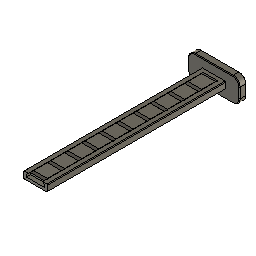
Price Tracker Final (Autodesk Fusion 360 design; units mm, degrees)
Autodesk Fusion 360 part; units mm, degrees
sketch "Sketch1" plane through (0, 0, 0) normal (0, 0, 1) x (1, 0, 0)
  line L0 (12.5, -12.5) -> (-12.5, -12.5)
  line L1 (-12.5, -12.5) -> (-12.5, 12.5)
  line L2 (-12.5, 12.5) -> (12.5, 12.5)
  line L3 (12.5, 12.5) -> (12.5, -12.5)
  line L4 (12.5, -12.5) -> (-12.5, 12.5) construction
  line L5 (-12.5, -12.5) -> (12.5, 12.5) construction
  dimension "d1" = 25
  dimension "d2" = 25
  constraint horizontal L0
  constraint perpendicular L0 L1
  constraint parallel L0 L2
  constraint parallel L1 L3
  constraint coincident L4 origin
  constraint coincident L5 origin
  measures "d1" distance of L1.end L2.end
  measures "d2" distance of L0.end L1.end
extrude "Extrude1" add sketch "Sketch1" along normal blind 5 makes body 1
chamfer "Chamfer1" distance 2.5 angle 45 1 faces at (4.1667, -4.1667, 5) on bodies 1
pattern_linear "R-Pattern1" count 10 spacing 25 along (0, 1, 0) of bodies 1 makes body 2 at (4.1667, 20.8333, 0) makes body 3 at (4.1667, 45.8333, 0) makes body 4 at (4.1667, 70.8333, 0) makes body 5 at (4.1667, 95.8333, 0) makes body 6 at (4.1667, 120.8333, 0) makes body 7 at (4.1667, 145.8333, 0) makes body 8 at (4.1667, 170.8333, 0) makes body 9 at (4.1667, 195.8333, 0) makes body 10 at (4.1667, 220.8333, 0)
sketch "Sketch2" plane through (0, 0, 0) normal (0, 0, 1) x (1, 0, 0)
  line L0 (17.5, 242.5) -> (-17.5, 242.5)
  line L1 (-17.5, 242.5) -> (-17.5, -17.5)
  line L2 (-17.5, -17.5) -> (17.5, -17.5)
  line L3 (17.5, -17.5) -> (17.5, 242.5)
  line L4 (17.5, 242.5) -> (-17.5, -17.5) construction
  line L5 (-17.5, 242.5) -> (17.5, -17.5) construction
  line L6 (-12.5, 12.5) -> (12.5, 12.5) construction
  line L7 (12.5, 12.5) -> (12.5, -12.5) construction
  line L8 (12.5, -12.5) -> (-12.5, -12.5) construction
  line L9 (-12.5, -12.5) -> (-12.5, 12.5) construction
  line L10 (-17.5, -17.5) -> (-17.5, 17.5)
  line L11 (-17.5, 17.5) -> (17.5, 17.5) construction
  line L12 (17.5, 17.5) -> (17.5, -17.5)
  line L13 (17.5, -17.5) -> (-17.5, -17.5)
  point P0 (0, 112.5)
  dimension "d11" = 35
  dimension "d12" = 260
  dimension "d13" = -5
  constraint horizontal L0
  constraint perpendicular L0 L1
  constraint parallel L0 L2
  constraint parallel L1 L3
  constraint coincident L4 P0
  constraint coincident L5 P0
  constraint coincident L1.end L2.start
  measures "d11" distance of L1.end L2.end
  measures "d12" distance of L0.end L1.end
extrude "Extrude2" add sketch "Sketch2" along normal blind 5 and the other way blind 5 separate body makes body 11
sketch "Sketch3" plane through (0, 0, 5) normal (0, 0, 1) x (-1, 0, 0)
  line L0 (-17.5, 17.5) -> (-17.5, -242.5)
  line L1 (17.5, -242.5) -> (17.5, 17.5)
  line L2 (13, -242.5) -> (13, 17.5)
  line L3 (-13, 17.5) -> (-13, -242.5)
  line L4 (17.5, 17.5) -> (-17.5, 17.5)
  line L5 (-17.5, -242.5) -> (17.5, -242.5)
  line L6 (-17.5, -237.5) -> (17.5, -237.5)
  dimension "d18" = -4.5
  dimension "d19" = -4.5
  dimension "d22" = 5
  constraint coincident L0 L6.start
  constraint coincident L1 L6.end
  constraint perpendicular L1 L6
  measures "d22" distance of L5 L6
extrude "Extrude3" cut sketch "Sketch3" against normal blind 6 contours L2 L3 L4 L6 bodies 11
sketch "Sketch4" plane through (0, -17.5, 0) normal (0, -1, 0) x (1, 0, 0)
  line L0 (13, 5) -> (13, -1)
  line L1 (13, -1) -> (-13, -1)
  line L2 (-13, -1) -> (-13, 5)
  line L3 (-13, 5) -> (-17.5, 5)
  line L4 (-17.5, 5) -> (-17.5, -5)
  line L5 (-17.5, -5) -> (17.5, -5)
  line L6 (17.5, -5) -> (17.5, 5)
  line L7 (17.5, 5) -> (13, 5)
  line L8 (13, 2.5) -> (10.5, 5)
  line L9 (10.5, 5) -> (13, 5)
  line L10 (0, 0) -> (0, 1.1872)
  line L11 (-13, 2.5) -> (-10.5, 5)
  line L12 (-10.5, 5) -> (-13, 5)
  dimension "d23" = 135
  dimension "d24" = 2.5
  dimension "d25" = 2.5
  constraint coincident L0 L8.start
  constraint coincident L0.start L7.end
  constraint coincident L10.start origin
  constraint perpendicular L1 L10
  constraint symmetric L8.start L10 L11.start
  constraint symmetric L8.end L10 L11.end
  constraint symmetric L0.start L10 L2.end
  measures "d23" angle of L0 L8
  measures "d24" distance of L8.end L0.start
  measures "d25" distance of L8.start L0.start
extrude "Extrude4" add sketch "Sketch4" against normal blind 255 contours L0 L8 L9 | L2 L11 L12 bodies 11
chamfer "Chamfer2" distance 1 angle 45 4 edges at (-17.5, 112.5, -5) (17.5, 112.5, 5) (-17.5, 112.5, 5) (17.5, 112.5, -5) on bodies 11
sketch "Sketch5" plane through (0, 242.5, 0) normal (0, 1, 0) x (-1, 0, 0)
  line L0 (-17.5, -4) -> (-16.5, -5)
  line L1 (-16.5, -5) -> (16.5, -5)
  line L2 (16.5, -5) -> (17.5, -4)
  line L3 (17.5, -4) -> (17.5, 4)
  line L4 (17.5, 4) -> (16.5, 5)
  line L5 (16.5, 5) -> (-16.5, 5)
  line L6 (-16.5, 5) -> (-17.5, 4)
  line L7 (-17.5, 4) -> (-17.5, -4)
  line L8 (37.5, -17.5) -> (-37.5, -17.5)
  line L9 (-37.5, -17.5) -> (-37.5, 17.5)
  line L10 (-37.5, 17.5) -> (37.5, 17.5)
  line L11 (37.5, 17.5) -> (37.5, -17.5)
  line L12 (37.5, -17.5) -> (-37.5, 17.5) construction
  line L13 (-37.5, -17.5) -> (37.5, 17.5) construction
  dimension "d29" = 75
  dimension "d30" = 35
  constraint horizontal L8
  constraint perpendicular L8 L9
  constraint parallel L8 L10
  constraint parallel L9 L11
  constraint coincident L12 origin
  constraint coincident L13 origin
  measures "d29" distance of L9.end L10.end
  measures "d30" distance of L8.end L9.end
extrude "Extrude5" add sketch "Sketch5" along normal blind 10 separate body contours L0 L1 L2 L3 L4 L5 L6 L7 | L8 L9 L10 L11 makes body 12
extrude "Extrude6" add 1 faces at (5.5, 242.5, -1.6667) along direction (0, 1, 0) blind 10 on bodies 11 bodies 11
combine "Combine2" operation cut target body 12 tool bodies 11 keep tools
sketch "Sketch6" plane through (0, 252.5, 0) normal (0, 1, 0) x (-1, 0, 0)
  line L0 (16.5, 5) -> (17.5, 4)
  line L1 (17.5, 4) -> (17.5, -4)
  line L2 (17.5, -4) -> (16.5, -5)
  line L3 (16.5, -5) -> (-16.5, -5)
  line L4 (-16.5, -5) -> (-17.5, -4)
  line L5 (-17.5, -4) -> (-17.5, 4)
  line L6 (-17.5, 4) -> (-16.5, 5)
  line L7 (-16.5, 5) -> (16.5, 5)
  line L8 (37.5, -17.5) -> (37.5, 17.5)
  line L9 (37.5, 17.5) -> (-37.5, 17.5)
  line L10 (-37.5, 17.5) -> (-37.5, -17.5)
  line L11 (-37.5, -17.5) -> (37.5, -17.5)
  line L12 (-16.5414, 5.1) -> (16.5414, 5.1)
  line L13 (16.5414, 5.1) -> (17.6, 4.0414)
  line L14 (17.6, 4.0414) -> (17.6, -4.0414)
  line L15 (17.6, -4.0414) -> (16.5414, -5.1)
  line L16 (16.5414, -5.1) -> (-16.5414, -5.1)
  line L17 (-16.5414, -5.1) -> (-17.6, -4.0414)
  line L18 (-17.6, -4.0414) -> (-17.6, 4.0414)
  line L19 (-17.6, 4.0414) -> (-16.5414, 5.1)
  dimension "d36" = -0.1
extrude "Extrude7" cut sketch "Sketch6" against normal blind 10 contours L12 L13 L14 L15 L16 L17 L18 L19 bodies 12
fillet "Fillet1" radius 10 4 edges at (37.5, 247.5, 17.5) (37.5, 247.5, -17.5) (-37.5, 247.5, 17.5) (-37.5, 247.5, -17.5) on bodies 12
chamfer "Chamfer4" distance 1 angle 45 16 edges at (0, 252.5, 17.5) (34.5711, 252.5, 14.5711) (37.5, 252.5, 0) (34.5711, 252.5, -14.5711) (0, 252.5, -17.5) (-34.5711, 252.5, -14.5711) (-37.5, 252.5, 0) (-34.5711, 252.5, 14.5711) (0, 242.5, 17.5) (-34.5711, 242.5, 14.5711) (-37.5, 242.5, 0) (-34.5711, 242.5, -14.5711) (0, 242.5, -17.5) (34.5711, 242.5, -14.5711) (37.5, 242.5, 0) (34.5711, 242.5, 14.5711) on bodies 12
equation "d7 = NumberOfPins"
equation "d12 = ( 25 * NumberOfPins ) * 1 mm + 10 mm"
equation "d26 = ( -25 * NumberOfPins ) * 1 mm - 5 mm"
equation "NumberOfPins = 10"
named bodies: "Body", "Base"
